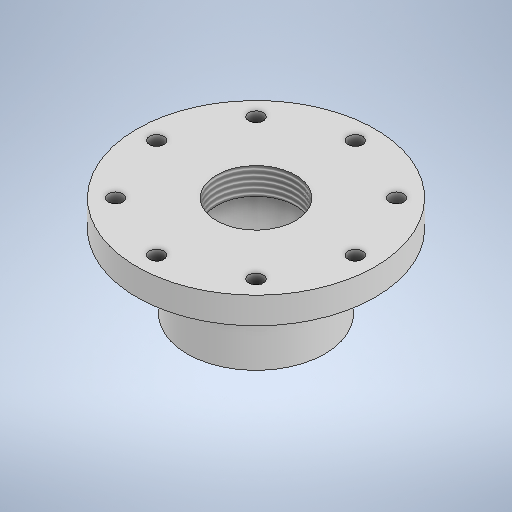
# Autodesk Inventor part: Passthrough Base
Saved by Autodesk Inventor 2025 (Build 290162000, 162)
## iProperties
Created: 2024-04-16
Part Number: Passthrough Base
Material: Generic
Document SubType Name: Modeling
Designer: cfang
Density: 1 g/cm^3
Appearance: Default
Author: cfang
Autodesk Inventor part; units mm, degrees
ref_plane "YZ Plane" through (0, 0, 0) normal (1, 0, 0) x (0, 1, 0)
ref_plane "XZ Plane" through (0, 0, 0) normal (0, 1, 0) x (-1, 0, 0)
ref_plane "XY Plane" through (0, 0, 0) normal (0, 0, 1) x (1, 0, 0)
sketch "Sketch1" plane through (0, 0, 0) normal (0, 1, 0) x (-1, 0, 0)
  circle A0 centre (0, 0) radius 45
  dimension "d0" = 90
  constraints: 1 centre point, 1 coincident
  measures "d0" diameter of A0
extrude "Extrusion1" add sketch "Sketch1" along normal blind 10
sketch "Sketch2" plane through (0, 0, 0) normal (0, -1, 0) x (1, 0, 0)
  circle A0 centre (0, 0) radius 26
  dimension "d3" = 52
  constraints: 1 centre point, 1 coincident
  measures "d3" diameter of A0
extrude "Extrusion2" add sketch "Sketch2" along normal blind 28
sketch "Sketch3" plane through (0, -28, 0) normal (0, -1, 0) x (1, 0, 0)
  circle A0 centre (0, 0) radius 21
  dimension "d6" = 42
  constraints: 1 centre point, 1 coincident
  measures "d6" diameter of A0
extrude "Extrusion3" cut sketch "Sketch3" against normal blind 28
sketch "Sketch4" plane through (0, -28, 0) normal (0, -1, 0) x (1, 0, 0)
  circle A0 centre (0, 0) radius 22.1
  circle A1 centre (0, 0) radius 24.8
  dimension "d9" = 44.2
  dimension "d10" = 49.6
  constraints: 2 centre point, 2 coincident
  measures "d9" diameter of A0
  measures "d10" diameter of A1
extrude "Extrusion4" cut sketch "Sketch4" against normal blind 2.2
sketch "Sketch5" plane through (0, 0, 0) normal (0, -1, 0) x (1, 0, 0)
  point P0 (0, 0)
  point P1 (0, 0)
  constraints: 1 coincident
hole "Hole1" at (0, 0, 0) direction (0, 1, 0) diameter 29.8349 end through all thread size "M32x2" class "6H" standard "ANSI Metric M Profile"
sketch "Sketch6" plane through (0, 0, 0) normal (0, -1, 0) x (1, 0, 0)
  point P0 (0, 0)
  point P1 (0, 37.5)
  point P2 (-26.5165, 26.5165)
  point P3 (-37.5, 0)
  point P4 (-26.5165, -26.5165)
  point P5 (0, -37.5)
  point P6 (26.5165, -26.5165)
  point P7 (37.5, 0)
  point P8 (26.5165, 26.5165)
  dimension "d20" = 37.5
  dimension "d30" = 360
  constraints: 9 other
  measures "d20" distance of point (0, 37.5) point (0, 0)
hole "Hole2" at (0, 0, 37.5) at (-26.5165, 0, 26.5165) at (-37.5, 0, 0) at (-26.5165, 0, -26.5165) at (0, 0, -37.5) at (26.5165, 0, -26.5165) at (37.5, 0, 0) at (26.5165, 0, 26.5165) direction (0, 1, 0) diameter 5.5 end through all countersink diameter 10.4 countersink angle 90 clearance for "Flat Head Machine Screw" size "M5" standard "Ansi Metric M Profile"
body "Solid1"
